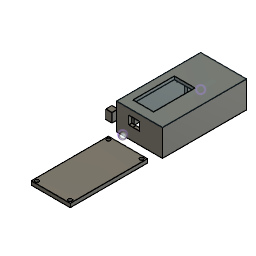
cover (Autodesk Fusion 360 design; units mm, degrees)
part number: 2026-06-01-12-34-53-255
Autodesk Fusion 360 part; units mm, degrees
sketch "Sketch1" plane through (0, 0, 0) normal (0, 1, 0) x (1, 0, 0)
  line L0 (0, 0) -> (-4, 0)
  line L1 (-4, 0) -> (-4, 110)
  line L2 (-4, 110) -> (0, 110)
  line L3 (0, 110) -> (0, 0)
  dimension "d1" = 4
  dimension "d2" = 110
  constraint horizontal L0
  constraint vertical L1
  constraint horizontal L2
  constraint vertical L3
  constraint coincident L0.start L3.end
  measures "d1" distance of L0.start L0.end
  measures "d2" distance of L0.start L2.end
extrude "Extrude1" add sketch "Sketch1" along normal blind 29 makes body 1
extrude "Extrude2" add 1 faces at (-1.3333, 29, -36.6667) along direction (0, 1, 0) blind 1 on bodies 1 bodies 1
sketch "Sketch2" plane through (0, 0, 0) normal (1, 0, 0) x (0, 0, -1)
  line L0 (0, 0) -> (110, 0)
  line L1 (110, 0) -> (110, 30)
  line L2 (110, 30) -> (0, 30)
  line L3 (0, 30) -> (0, 0)
  line L4 (0, 30) -> (4, 30)
  line L5 (4, 30) -> (4, 0)
  line L6 (4, 0) -> (0, 0)
  line L7 (0, 0) -> (0, 30)
  constraint horizontal L4
  constraint vertical L5
  constraint horizontal L6
  constraint vertical L7
  constraint coincident L0 L5.end
  constraint coincident L2.end L3.start
extrude "Extrude3" add sketch "Sketch2" along normal blind 56 contours L0 L2 L3 L4 L5 L6 L7 bodies 1
extrude "Extrude4" add 1 faces at (-2.6667, 30, -38) along direction (0, 1, 0) blind 5 on bodies 1 bodies 1
sketch "Sketch3" plane through (0, 0, 0) normal (1, 0, 0) x (0, 0, -1)
  line L0 (4, 35) -> (4, 0)
  line L1 (4, 0) -> (110, 0)
  line L2 (110, 0) -> (110, 35)
  line L3 (110, 35) -> (4, 35)
  line L4 (110, 35) -> (106, 35)
  line L5 (106, 35) -> (106, 0)
  line L6 (106, 0) -> (110, 0)
  line L7 (110, 0) -> (110, 35)
  constraint horizontal L4
  constraint vertical L5
  constraint horizontal L6
  constraint vertical L7
  constraint coincident L1 L5.end
  constraint coincident L2.end L3.start
extrude "Extrude5" add sketch "Sketch3" along normal blind 56 contours L1 L2 L3 L4 L5 L6 L7 bodies 1
sketch "Sketch4" plane through (0, 0, 0) normal (1, 0, 0) x (0, 0, -1)
  line L0 (106, 0) -> (106, 35)
  line L1 (106, 35) -> (4, 35)
  line L2 (4, 35) -> (4, 0)
extrude "Extrude6" add 1 faces at (-2.6667, 35, -72) along direction (0, 1, 0) blind 3 on bodies 1 bodies 1
sketch "Sketch5" plane through (0, 0, 0) normal (1, 0, 0) x (0, 0, -1)
  line L0 (106, 38) -> (4, 38)
  line L1 (4, 38) -> (4, 34)
  line L2 (4, 34) -> (106, 34)
  line L3 (106, 34) -> (106, 38)
  dimension "d15" = 102
  dimension "d16" = 4
  constraint horizontal L0
  constraint vertical L1
  constraint horizontal L2
  constraint vertical L3
  measures "d15" distance of L0.start L0.end
  measures "d16" distance of L0.start L2.end
extrude "Extrude7" add sketch "Sketch5" along normal blind 56 bodies 1
sketch "Sketch6" plane through (0, 38, 0) normal (0, 1, 0) x (-1, 0, 0)
  line L0 (-56, -110) -> (4, -110)
  line L1 (4, -110) -> (4, 0)
  line L2 (4, 0) -> (-56, 0)
  line L3 (-56, 0) -> (-56, -110)
  line L4 (-56, 0) -> (-56, -5)
  line L5 (4, -5) -> (-1, -5)
  line L6 (-1, -5) -> (-1, -110)
  line L7 (-1, -110) -> (-1, -105)
  line L8 (-56, -105) -> (-51, -105)
  line L9 (-51, -105) -> (-1, -105)
  line L10 (-51, -105) -> (-51, -5)
  line L11 (-51, -5) -> (-1, -5)
  line L12 (-1, -5) -> (-1, -12)
  line L13 (-1, -12) -> (-7, -12)
  line L14 (-7, -12) -> (-32, -12)
  line L15 (-32, -12) -> (-33, -12)
  line L16 (-33, -12) -> (-34, -12)
  line L17 (-34, -12) -> (-34, -66)
  line L18 (-34, -66) -> (0, -66)
  dimension "d19" = 25
  dimension "d20" = 54
  constraint coincident L2.end L3.start
  constraint coincident L3 L4.end
  constraint coincident L1 L5.start
  constraint perpendicular L1 L5
  constraint coincident L0 L6.end
  constraint perpendicular L0 L6
  constraint coincident L6 L7.end
  constraint coincident L3 L8.start
  constraint perpendicular L3 L8
  constraint perpendicular L6 L9
  constraint perpendicular L2 L10
  constraint perpendicular L6 L11
  constraint coincident L6 L12.end
  constraint perpendicular L6 L13
  constraint perpendicular L6 L14
  constraint perpendicular L1 L15
  constraint perpendicular L1 L16
  constraint perpendicular L16 L17
  constraint perpendicular L6 L18
  measures "d19" distance of L13.end L14.end
  measures "d20" distance of L16.end L17.end
extrude "Extrude8" cut sketch "Sketch6" against normal blind 30 contours L6 L13 L14 L15 L16 L17 L18 bodies 1
sketch "Sketch7" plane through (0, 34, 0) normal (0, -1, 0) x (1, 0, 0)
  line L0 (34, -12) -> (34, -66)
  line L1 (34, -66) -> (1, -66)
  line L2 (1, -66) -> (1, -12)
  line L3 (1, -12) -> (34, -12)
  line L4 (0, -4) -> (0, -106)
  line L5 (0, -106) -> (56, -106)
  line L6 (56, -106) -> (56, -4)
  line L7 (56, -4) -> (0, -4)
  line L8 (1, -69) -> (15.5, -69)
  line L9 (15.5, -69) -> (15.5, -106)
  line L10 (15.5, -69) -> (20, -69)
  line L11 (20, -69) -> (20, -106)
  line L12 (15.5, -106) -> (20, -106)
  constraint perpendicular L4 L8
  constraint coincident L5 L9.end
  constraint perpendicular L5 L9
  constraint perpendicular L9 L10
  constraint coincident L5 L11.end
  constraint perpendicular L5 L11
extrude "Extrude9" add sketch "Sketch7" along normal blind 15 contours L5 L9 L10 L11 L12 bodies 1
extrude "Extrude10" add 1 faces at (-2.6667, 0, -38) along direction (0, -1, 0) blind 2 on bodies 1 bodies 1
sketch "Sketch8" plane through (0, 0, 0) normal (1, 0, 0) x (0, 0, -1)
  line L0 (4, -2) -> (5, -2)
  line L1 (5, -2) -> (5, -1)
  constraint horizontal L0
  constraint perpendicular L0 L1
fillet "Fillet1" radius 1.5 1 edges at (20, 34, -87.5) on bodies 1
sketch "Sketch9" plane through (0, 0, 0) normal (1, 0, 0) x (0, 0, -1)
extrude "Extrude11" cut 1 faces at (-2.6667, -2, -38) along direction (0, 1, 0) blind 2 on bodies 1 bodies 1
extrude "Extrude12" cut 1 faces at (-2.6667, 0, -38) along direction (0, 1, 0) blind 2 on bodies 1 bodies 1
extrude "Extrude13" cut 1 faces at (-2.6667, 2, -38) along direction (0, 1, 0) blind 1 on bodies 1 bodies 1
sketch "Sketch10" plane through (0, 0, 0) normal (1, 0, 0) x (0, 0, -1)
  line L0 (4, 3) -> (106, 3)
  line L1 (106, 3) -> (106, 34)
  line L2 (106, 34) -> (4, 34)
  line L3 (4, 34) -> (4, 3)
  line L4 (5, 3) -> (5, 9)
  line L5 (5, 9) -> (5, 10)
  line L6 (5, 10) -> (105, 10)
  line L7 (105, 10) -> (105, 11)
  line L8 (105, 11) -> (5, 11)
  line L9 (5, 11) -> (5, 10)
  line L10 (102, 11) -> (102, 24)
  line L11 (102, 24) -> (102, 32)
  line L12 (102, 32) -> (95, 32)
  line L13 (95, 32) -> (94, 32)
  line L14 (94, 32) -> (94, 24)
  line L15 (94, 24) -> (102, 24)
  constraint coincident L0 L4.start
  constraint perpendicular L0 L4
  constraint perpendicular L5 L6
  constraint perpendicular L6 L7
  constraint perpendicular L3 L8
  constraint perpendicular L6 L9
  constraint coincident L8 L10.start
  constraint perpendicular L8 L10
  constraint perpendicular L8 L11
  constraint perpendicular L11 L12
  constraint perpendicular L11 L13
  constraint perpendicular L13 L14
  constraint perpendicular L11 L15
extrude "Extrude14" cut sketch "Sketch10" against normal blind 41 contours L11 L12 L13 L14 L15 bodies 1
extrude "Extrude15" add 1 faces at (-1.3333, 29.3333, -94) along direction (0, 0, -1) blind 1 on bodies 1 bodies 1
extrude "Extrude16" add 1 faces at (-1.3333, 32, -99.6667) along direction (0, -1, 0) blind 1 on bodies 1 bodies 1
sketch "Sketch11" plane through (0, 0, 0) normal (1, 0, 0) x (0, 0, -1)
  line L0 (102, 31) -> (102, 24)
  line L1 (102, 24) -> (95, 24)
  line L2 (95, 24) -> (95, 31)
  line L3 (95, 31) -> (102, 31)
  line L4 (4, 3) -> (106, 3)
  line L5 (106, 3) -> (106, 34)
  line L6 (106, 34) -> (4, 34)
  line L7 (4, 34) -> (4, 3)
  line L8 (5, 3) -> (5, 11)
  line L9 (5, 11) -> (105, 11)
  line L10 (105, 11) -> (105, 12)
  line L11 (105, 12) -> (5, 12)
  line L12 (5, 12) -> (5, 11)
  line L13 (105, 12) -> (83, 12)
  line L14 (83, 12) -> (83, 24)
  line L15 (83, 24) -> (75, 24)
  line L16 (75, 24) -> (75, 32)
  line L17 (75, 32) -> (83, 32)
  line L18 (83, 32) -> (83, 24)
  constraint coincident L4 L8.start
  constraint perpendicular L4 L8
  constraint perpendicular L5 L9
  constraint perpendicular L9 L10
  constraint perpendicular L10 L11
  constraint perpendicular L9 L12
  constraint coincident L11 L13.end
  constraint perpendicular L1 L14
  constraint perpendicular L14 L15
  constraint perpendicular L15 L16
  constraint perpendicular L16 L17
  constraint perpendicular L15 L18
extrude "Extrude17" cut sketch "Sketch11" against normal blind 21 contours L15 L16 L17 L18 bodies 1
extrude "Extrude18" cut 1 faces at (-1.3333, 31, -99.6667) along direction (0, 1, 0) blind 1 on bodies 1 bodies 1
extrude "Extrude19" cut 1 faces at (-1.3333, 29.3333, -95) along direction (0, 0, 1) blind 1 on bodies 1 bodies 1
sketch "Sketch12" plane through (0, 38, 0) normal (0, 1, 0) x (-1, 0, 0)
  line L0 (-56, -110) -> (4, -110)
  line L1 (4, -110) -> (4, 0)
  line L2 (4, 0) -> (-56, 0)
  line L3 (-56, 0) -> (-56, -110)
sketch "Sketch13" plane through (0, 0, 0) normal (0, 0, 1) x (1, 0, 0)
  line L0 (-4, 3) -> (56, 3)
  line L1 (56, 3) -> (56, 38)
  line L2 (56, 38) -> (-4, 38)
  line L3 (-4, 38) -> (-4, 3)
  line L4 (17.5, 3) -> (17.5, 11)
  line L5 (17.5, 11) -> (17.5, 19)
  line L6 (17.5, 19) -> (24.5, 19)
  line L7 (24.5, 19) -> (24.5, 20.1)
  line L8 (24.5, 19) -> (24.5, 30)
  line L9 (24.5, 30) -> (10.5, 30)
  line L10 (10.5, 30) -> (10.5, 19)
  line L11 (10.5, 19) -> (17.5, 19)
  dimension "d48" = 8
  dimension "d49" = 7
  dimension "d50" = 1.1
  dimension "d51" = 11
  dimension "d52" = 14
  constraint coincident L0 L4.start
  constraint perpendicular L0 L4
  constraint perpendicular L0 L5
  constraint perpendicular L5 L6
  constraint perpendicular L6 L7
  constraint perpendicular L6 L8
  constraint perpendicular L8 L9
  constraint perpendicular L9 L10
  measures "d48" distance of L4.end L5.end
  measures "d49" distance of L5.end L6.end
  measures "d50" distance of L6.end L7.end
  measures "d51" distance of L6.end L8.end
  measures "d52" distance of L8.end L9.end
extrude "Extrude20" cut sketch "Sketch13" against normal blind 20 contours L6 L7 L8 L9 L10 L11 bodies 1
extrude "Extrude21" add 1 faces at (1, 36.6667, -30) along direction (1, 0, 0) blind 6 on bodies 1 bodies 1
extrude "Extrude22" cut 1 faces at (24.5, 22.6667, -1.3333) along direction (1, 0, 0) blind 6 on bodies 1 bodies 1
extrude "Extrude23" cut 1 faces at (7, 36.6667, -30) along direction (-1, 0, 0) blind 1 on bodies 1 bodies 1
extrude "Extrude24" cut 1 faces at (6, 36.6667, -30) along direction (-1, 0, 0) blind 0.5 on bodies 1 bodies 1
extrude "Extrude25" add 1 faces at (34, 36.6667, -30) along direction (-1, 0, 0) blind 1.5 on bodies 1 bodies 1
sketch "Sketch14" plane through (0, 38, 0) normal (0, 1, 0) x (-1, 0, 0)
extrude "Extrude26" add 1 faces at (30.5, 22.6667, -1.3333) along direction (-1, 0, 0) blind 3 on bodies 1 bodies 1
extrude "Extrude27" add 1 faces at (10.5, 26.3333, -1.3333) along direction (1, 0, 0) blind 1 on bodies 1 bodies 1
extrude "Extrude28" add 1 faces at (27.5, 22.6667, -1.3333) along direction (-1, 0, 0) blind 1.5 on bodies 1 bodies 1
extrude "Extrude29" add 1 faces at (11.5, 26.3333, -1.3333) along direction (1, 0, 0) blind 0.5 on bodies 1 bodies 1
sketch "Sketch15" plane through (0, 34, 0) normal (0, -1, 0) x (1, 0, 0)
  line L0 (5.5, -12) -> (32.5, -12)
  line L1 (32.5, -12) -> (32.5, -66)
  line L2 (32.5, -66) -> (5.5, -66)
  line L3 (5.5, -66) -> (5.5, -12)
  line L4 (21.5, -69) -> (21.5, -106)
  line L5 (21.5, -106) -> (56, -106)
  line L6 (56, -106) -> (56, -4)
  line L7 (56, -4) -> (0, -4)
  line L8 (0, -4) -> (0, -106)
  line L9 (0, -106) -> (15.5, -106)
  line L10 (15.5, -106) -> (15.5, -69)
  line L11 (15.5, -69) -> (21.5, -69)
  line L12 (56, -4) -> (52, -4)
  line L13 (52, -4) -> (52, -106)
  line L14 (52, -106) -> (56, -106)
  line L15 (56, -106) -> (56, -4)
  dimension "d73" = 4
  constraint horizontal L12
  constraint vertical L13
  constraint horizontal L14
  constraint vertical L15
  constraint coincident L5 L13.end
  constraint coincident L6.end L7.start
  measures "d73" distance of L6.end L12.end
extrude "Extrude30" add sketch "Sketch15" along normal blind 31 contours L5 L6 L7 L12 L13 L14 L15 bodies 1
sketch "Sketch16" plane through (0, 19, 0) normal (0, -1, 0) x (1, 0, 0)
  line L0 (15.5, -69) -> (15.5, -106)
  line L1 (15.5, -106) -> (20, -106)
  line L2 (20, -106) -> (20, -69)
  line L3 (20, -69) -> (15.5, -69)
sketch "Sketch17" plane through (0, 34, 0) normal (0, -1, 0) x (1, 0, 0)
  line L0 (52, -106) -> (52, -4)
  line L1 (52, -4) -> (0, -4)
  line L2 (0, -4) -> (0, -106)
  line L3 (0, -106) -> (15.5, -106)
  line L4 (15.5, -106) -> (15.5, -69)
  line L5 (15.5, -69) -> (21.5, -69)
  line L6 (21.5, -69) -> (21.5, -106)
  line L7 (21.5, -106) -> (52, -106)
  line L8 (5.5, -12) -> (32.5, -12)
  line L9 (32.5, -12) -> (32.5, -66)
  line L10 (32.5, -66) -> (5.5, -66)
  line L11 (5.5, -66) -> (5.5, -12)
  line L12 (52, -4) -> (44.5, -4)
  line L13 (44.5, -4) -> (44.5, -11.5)
  line L14 (44.5, -11.5) -> (52, -11.5)
  line L15 (52, -4) -> (52, -11.5)
  dimension "d76" = 7.5
  constraint coincident L0.end L1.start
  constraint coincident L1 L12.end
  constraint perpendicular L12 L13
  constraint coincident L0 L14.end
  constraint perpendicular L0 L14
  measures "d76" distance of L12.end L13.end
extrude "Extrude31" add sketch "Sketch17" along normal blind 22.5 contours L0 L1 L12 L13 L14 L15 bodies 1
sketch "Sketch18" plane through (0, 34, 0) normal (0, -1, 0) x (1, 0, 0)
  line L0 (5.5, -12) -> (32.5, -12)
  line L1 (32.5, -12) -> (32.5, -66)
  line L2 (32.5, -66) -> (5.5, -66)
  line L3 (5.5, -66) -> (5.5, -12)
  line L4 (52, -11.5) -> (44.5, -11.5)
  line L5 (44.5, -11.5) -> (44.5, -4)
  line L6 (44.5, -4) -> (0, -4)
  line L7 (0, -4) -> (0, -106)
  line L8 (0, -106) -> (15.5, -106)
  line L9 (15.5, -106) -> (15.5, -69)
  line L10 (15.5, -69) -> (21.5, -69)
  line L11 (21.5, -69) -> (21.5, -106)
  line L12 (21.5, -106) -> (52, -106)
  line L13 (52, -106) -> (52, -11.5)
  line L14 (52, -106) -> (44.5, -106)
  line L15 (44.5, -106) -> (44.5, -98.5)
  line L16 (44.5, -98.5) -> (52, -98.5)
  line L17 (52, -98.5) -> (52, -106)
  dimension "d79" = 7.5
  dimension "d80" = 7.5
  constraint horizontal L14
  constraint vertical L15
  constraint horizontal L16
  constraint vertical L17
  constraint coincident L12.end L13.start
  measures "d79" distance of L12.end L14.end
  measures "d80" distance of L12.end L16.end
extrude "Extrude32" add sketch "Sketch18" along normal blind 22.5 contours L12 L13 L14 L15 L16 L17 bodies 1
sketch "Sketch19" plane through (0, 34, 0) normal (0, -1, 0) x (1, 0, 0)
  line L0 (44.5, -106) -> (44.5, -98.5)
  line L1 (44.5, -98.5) -> (52, -98.5)
  line L2 (52, -98.5) -> (52, -11.5)
  line L3 (52, -11.5) -> (44.5, -11.5)
  line L4 (44.5, -11.5) -> (44.5, -4)
  line L5 (44.5, -4) -> (0, -4)
  line L6 (0, -4) -> (0, -106)
  line L7 (0, -106) -> (15.5, -106)
  line L8 (15.5, -106) -> (15.5, -69)
  line L9 (15.5, -69) -> (21.5, -69)
  line L10 (21.5, -69) -> (21.5, -106)
  line L11 (21.5, -106) -> (44.5, -106)
  line L12 (5.5, -12) -> (32.5, -12)
  line L13 (32.5, -12) -> (32.5, -66)
  line L14 (32.5, -66) -> (5.5, -66)
  line L15 (5.5, -66) -> (5.5, -12)
  line L16 (0, -4) -> (7.5, -4)
  line L17 (7.5, -4) -> (7.5, -11.5)
  line L18 (7.5, -11.5) -> (0, -11.5)
  line L19 (0, -11.5) -> (0, -4)
  dimension "d83" = 7.5
  dimension "d84" = 7.5
  constraint horizontal L16
  constraint vertical L17
  constraint horizontal L18
  constraint vertical L19
  constraint coincident L5.end L6.start
  measures "d83" distance of L5.end L16.end
  measures "d84" distance of L5.end L18.end
extrude "Extrude33" add sketch "Sketch19" along normal blind 22.5 contours L5 L6 L16 L17 L18 L19 bodies 1
sketch "Sketch20" plane through (0, 3, 0) normal (0, -1, 0) x (1, 0, 0)
  line L0 (52, -106) -> (0, -106)
  line L1 (0, -106) -> (0, -4)
  line L2 (0, -4) -> (52, -4)
  line L3 (52, -4) -> (52, -106)
  line L4 (56, -110) -> (56, 0)
  line L5 (56, 0) -> (-4, 0)
  line L6 (-4, 0) -> (-4, -110)
  line L7 (-4, -110) -> (56, -110)
  line L8 (0.5, 5) -> (51.5, 5)
  line L9 (51.5, 5) -> (51.5, 106)
  line L10 (51.5, 106) -> (0.5, 106)
  line L11 (0.5, 106) -> (0.5, 5)
  dimension "d87" = 101
  constraint parallel L5 L8
  constraint perpendicular L0 L9
  constraint perpendicular L9 L10
  constraint perpendicular L8 L11
  measures "d87" distance of L8.end L9.end
extrude "Extrude34" add sketch "Sketch20" against normal blind 5 separate body contours L8 L9 L10 L11 makes body 2
sketch "Sketch21" plane through (0, 11.5, 0) normal (0, -1, 0) x (1, 0, 0)
  line L0 (52, -98.5) -> (44.5, -98.5)
  line L1 (44.5, -98.5) -> (44.5, -106)
  line L2 (44.5, -106) -> (52, -106)
  line L3 (52, -106) -> (52, -98.5)
  circle A0 centre (4, -7.5) radius 2
extrude "Extrude35" cut sketch "Sketch21" against normal blind 7 contours A0 bodies 1
sketch "Sketch22" plane through (0, 11.5, 0) normal (0, -1, 0) x (1, 0, 0)
  circle A0 centre (4, -7.5) radius 2
  line L0 (0, -11.5) -> (7.5, -11.5)
  line L1 (7.5, -11.5) -> (7.5, -4)
  line L2 (7.5, -4) -> (0, -4)
  line L3 (0, -4) -> (0, -11.5)
extrude "Extrude36" add sketch "Sketch22" along normal blind 7 separate body contours A0 makes body 3
sketch "Sketch23" plane through (0, 4.5, 0) normal (0, -1, 0) x (1, 0, 0)
  circle A0 centre (4, -7.5) radius 2
extrude "Extrude37" cut sketch "Sketch23" against normal blind 7 bodies 3
extrude "Extrude38" add 1 faces at (4.7854, 18.5, -7.0466) along direction (0, -1, 0) blind 7 on bodies 1 bodies 1 3
sketch "Sketch24" plane through (0, 11.5, 0) normal (0, -1, 0) x (1, 0, 0)
  line L0 (0, -11.5) -> (7.5, -11.5)
  line L1 (7.5, -11.5) -> (7.5, -4)
  line L2 (7.5, -4) -> (0, -4)
  line L3 (0, -4) -> (0, -11.5)
  line L4 (0, -4) -> (2, -4)
  line L5 (2, -4) -> (2, -6)
  line L6 (2, -6) -> (3, -7)
  circle A0 centre (3.5, -7.5) radius 2
  constraint coincident L2.end L3.start
  constraint coincident L2 L4.end
  constraint perpendicular L2 L5
extrude "Extrude39" cut sketch "Sketch24" against normal blind 7 contours A0 bodies 1
sketch "Sketch25" plane through (0, 11.5, 0) normal (0, -1, 0) x (1, 0, 0)
  line L0 (44.5, -4) -> (44.5, -11.5)
  line L1 (44.5, -11.5) -> (52, -11.5)
  line L2 (52, -11.5) -> (52, -4)
  line L3 (52, -4) -> (44.5, -4)
  circle A0 centre (48.5, -7.5) radius 2
extrude "Extrude40" cut sketch "Sketch25" against normal blind 7 contours A0 bodies 1
sketch "Sketch26" plane through (0, 11.5, 0) normal (0, -1, 0) x (1, 0, 0)
  line L0 (52, -98.5) -> (44.5, -98.5)
  line L1 (44.5, -98.5) -> (44.5, -106)
  line L2 (44.5, -106) -> (52, -106)
  line L3 (52, -106) -> (52, -98.5)
  circle A0 centre (48.5, -102.5) radius 2
extrude "Extrude41" cut sketch "Sketch26" against normal blind 7 contours A0 bodies 1
sketch "Sketch27" plane through (0, 3, 0) normal (0, -1, 0) x (1, 0, 0)
  line L0 (0.5, 106) -> (0.5, 5)
  line L1 (0.5, 5) -> (51.5, 5)
  line L2 (51.5, 5) -> (51.5, 106)
  line L3 (51.5, 106) -> (0.5, 106)
  circle A0 centre (4.2885, 8.7885) radius 2.4205
extrude "Extrude42" add sketch "Sketch27" along normal blind 7 contours A0 bodies 2
extrude "Extrude43" cut 1 faces at (3.579, -4, 10.0883) along direction (0, 1, 0) blind 14 on bodies 2 bodies 2
sketch "Sketch28" plane through (0, 3, 0) normal (0, -1, 0) x (1, 0, 0)
  circle A0 centre (4.2885, 8.7885) radius 2.4205
  line L0 (0.5, 106) -> (0.5, 5)
  line L1 (0.5, 5) -> (51.5, 5)
  line L2 (51.5, 5) -> (51.5, 106)
  line L3 (51.5, 106) -> (0.5, 106)
  circle A1 centre (47.7115, 8.7885) radius 2.4205
extrude "Extrude44" cut sketch "Sketch28" against normal blind 7 contours A1 bodies 2
sketch "Sketch29" plane through (0, 3, 0) normal (0, -1, 0) x (1, 0, 0)
  circle A0 centre (47.7115, 8.7885) radius 2.4205
  circle A1 centre (4.2885, 8.7885) radius 2.4205
  line L0 (0.5, 106) -> (0.5, 5)
  line L1 (0.5, 5) -> (51.5, 5)
  line L2 (51.5, 5) -> (51.5, 106)
  line L3 (51.5, 106) -> (0.5, 106)
  circle A2 centre (47.7115, 102.2115) radius 2.4205
extrude "Extrude45" cut sketch "Sketch29" against normal blind 7 contours A2 bodies 2
sketch "Sketch30" plane through (0, 3, 0) normal (0, -1, 0) x (1, 0, 0)
  circle A0 centre (47.7115, 102.2115) radius 2.4205
  circle A1 centre (47.7115, 8.7885) radius 2.4205
  circle A2 centre (4.2885, 8.7885) radius 2.4205
  line L0 (0.5, 106) -> (0.5, 5)
  line L1 (0.5, 5) -> (51.5, 5)
  line L2 (51.5, 5) -> (51.5, 106)
  line L3 (51.5, 106) -> (0.5, 106)
  circle A3 centre (4.2885, 102.2115) radius 2.4205
extrude "Extrude46" add sketch "Sketch30" along normal blind 76 contours A3 bodies 2
extrude "Extrude47" cut 1 faces at (5.0757, -73, 102.666) along direction (0, 1, 0) blind 7 on bodies 2 bodies 2
extrude "Extrude48" cut 1 faces at (5.0757, -66, 102.666) along direction (0, 1, 0) blind 7 on bodies 2 bodies 2
extrude "Extrude49" cut 1 faces at (5.0757, -59, 102.666) along direction (0, 1, 0) blind 100000 on bodies 2 bodies 2
sketch "Sketch31" plane through (0, 0, 0) normal (0, 1, 0) x (1, 0, 0)
  line L0 (-20, 10) -> (-28, 10)
  line L1 (-28, 10) -> (-28, 18)
  line L2 (-28, 18) -> (-20, 18)
  line L3 (-20, 18) -> (-20, 10)
  dimension "d120" = 8
  dimension "d121" = 8
  constraint horizontal L0
  constraint vertical L1
  constraint horizontal L2
  constraint vertical L3
  measures "d120" distance of L0.start L0.end
  measures "d121" distance of L0.start L2.end
extrude "Extrude50" add sketch "Sketch31" along normal blind 12 separate body makes body 4
copy_body "CopyPasteBodies1" bodies 4 makes body 5
move_body "Move1" bodies 5 to x (1, 0, 0) y (0, 1, 0) z (0, 0, 1) at (0, 0, -15)
move_face "MoveFace1" by (0, 0, 15) 1 faces at (19.0576, 8, 70.3195) on bodies 2
move_body "Move2" bodies 2 to x (1, 0, 0) y (0, 1, 0) z (0, 0, 1) at (0, 0, 10)
